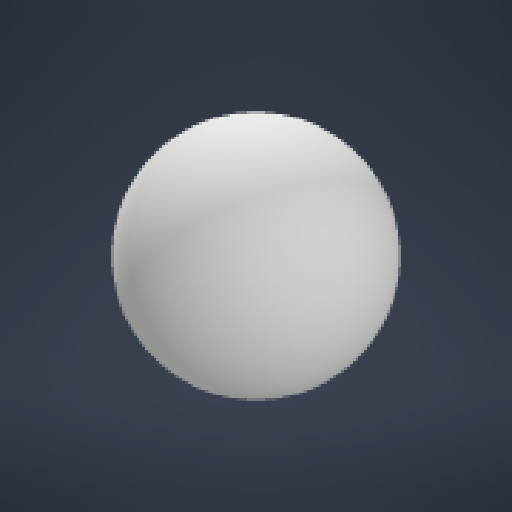
# Autodesk Inventor part: roll_ball_1
Saved by Autodesk Inventor 2026 (Build 300175050, 175E)
## iProperties
Created: 2026-04-01
Part Number: roll_ball_1
Material: Generic
Document SubType Name: Modeling
Designer: sniel
Density: 1 g/cm^3
Appearance: Default
Author: sniel
Autodesk Inventor part; units mm, degrees
ref_plane "YZ Plane" through (0, 0, 0) normal (1, 0, 0) x (0, 1, 0)
ref_plane "XZ Plane" through (0, 0, 0) normal (0, 1, 0) x (-1, 0, 0)
ref_plane "XY Plane" through (0, 0, 0) normal (0, 0, 1) x (1, 0, 0)
sketch "Sketch1" plane through (0, 0, 0) normal (1, 0, 0) x (0, 1, 0)
  circle A0 centre (0, 0) radius 1.75
  line L0 (1.75, 0) -> (-1.75, 0)
  circle A1 centre (0, 0) radius 2.85
  line L1 (-2.85, 0) -> (2.85, 0)
  dimension "d3" = 5.7
  constraints: 4 end point, 4 point on circle, 2 centre point, 2 horizontal, 1 coincident
  measures "d3" diameter of A1
revolve "Revolution1" add sketch "Sketch1" angle 360 about axis through (0, 1.75, 0) along (0, -1, 0) picked at (2.4557, -0.2273) picked at (-0.3314, -0.4801) contours L1 A1 A0 | A0 L0
body "Solid1"
